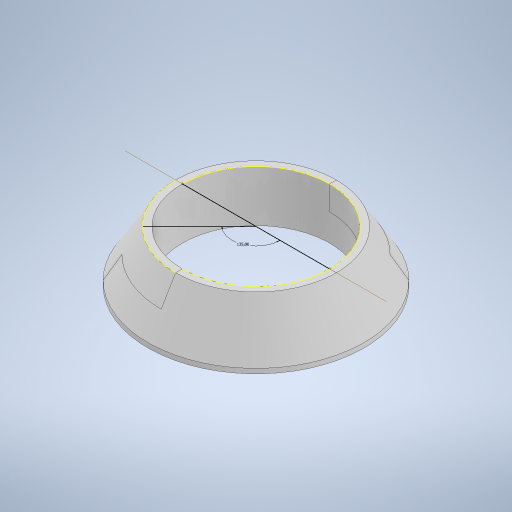
# Autodesk Inventor part: Kolanko
Saved by Autodesk Inventor 2024 (Build 280153000, 153)
## iProperties
Created: 2023-12-15
Part Number: Kolanko
Material: Generic
Document SubType Name: Modeling
Designer: Piter
Density: 1 g/cm^3
Appearance: Default
Author: Piter
Autodesk Inventor part; units mm, degrees
ref_plane "YZ Plane" through (0, 0, 0) normal (1, 0, 0) x (0, 1, 0)
sketch "Sketch1" plane through (0, 0, 0) normal (0, 1, 0) x (-1, 0, 0)
  circle A0 centre (0, 0) radius 27.25
  circle A1 centre (0, 0) radius 40
  line L0 (0, 0) -> (40, 0)
  line L1 (0, 0) -> (-40, 0)
  dimension "d0" = 54.5
  dimension "d1" = 80
  dimension "d2" = 12.75
  constraints: 4 end point, 2 centre point, 2 coincident, 2 point on circle, 1 horizontal
  measures "d0" diameter of A0
  measures "d1" diameter of A1
  measures "d2" radial gap between concentric circles of A1 A0
extrude "Extrusion1" add sketch "Sketch1" along normal blind 19 contours L0 A1 L1 A0 | A0 L1 A1 L0
chamfer "Chamfer2" distance 10.25 distance2 17.25 1 edges at (40, 19, 0) measured on face at (17.5776, 19, -30.8976)
ref_plane "Work Plane1" through (0, 10, 0) normal (0, 1, 0) x (-1, 0, 0)
split body "Split1" result two bodies by plane through (0, 10, 0) normal (0, 1, 0) first body at (-8.6629, 11.2446, 32.6469)
split body "Split2" result two bodies by plane through (0, 0, 0) normal (1, 0, 0) bodies 2 first body at (2.4575, 12.7446, 32.7934)
sketch "Sketch2" plane through (0, 19, 0) normal (0, 1, 0) x (1, 0, 0)
  arc A0 (0, 27.25) -> (-27.25, 0) centre (0, 0) ccw projected
  line L0 (-27.25, 0) -> (27.25, 0)
  arc A1 (0, -27.25) -> (0, 27.25) centre (0, 0) ccw projected
  line L1 (0, 0) -> (-21.0364, -21.0364)
  arc A2 (-29.75, 0) -> (0, -29.75) centre (0, 0) ccw projected
  line L2 (0, 0) -> (29.75, 0) construction
  dimension "d12" = 135
  constraints: 6 end point, 2 horizontal, 2 point on circle, 1 equal length
  measures "d12" angle of L1 L2
ref_plane "Work Plane2" through (0, 19, 0) normal (0.7071068, 0, 0.7071068) x (-0.7071068, 0, 0.7071068)
split body "Split3" result two bodies by plane through (0, 19, 0) normal (0.7071068, 0, 0.7071068) bodies 3 first body at (25.9031, 0.5, 24.3547)
combine bodies "Combine1" operation type add bodies to combine 6 4
combine bodies "Combine2" operation type add bodies to combine 7 5
body "Solid4"
body "Solid5"
